# Autodesk Inventor part: Shaft
Saved by Autodesk Inventor 2014 (Build 180170000, 170)
## iProperties
Created: 2014-08-25
Part Number: Shaft
Material: Steel
Document SubType Name: Modeling
Designer: sam
Density: 1 g/cm^3
Appearance: Steel
CustomPartVersion: 1
Author: sam
Autodesk Inventor part; units mm, degrees
ref_plane "Start Plane" through (0, 0, 0) normal (1, 0, 0) x (0, 1, 0)
ref_plane "XZ Plane" through (0, 0, 0) normal (0, 1, 0) x (-1, 0, 0)
ref_plane "XY Plane" through (0, 0, 0) normal (0, 0, 1) x (1, 0, 0)
sketch "Main Sketch" plane through (0, 0, 0) normal (0, 0, 1) x (1, 0, 0)
  line L0 (0, 0) -> (10, 0)
  line L1 (0, 0) -> (0, 5.912)
  line L2 (0, 5.912) -> (5, 5.912)
  line L3 (10, 5.912) -> (10, 0)
  line L4 (5, 5.912) -> (10, 5.912)
  dimension "d3" = 11.824
  dimension "d4" = 11.824
  constraints: 10 end point, 4 horizontal, 2 vertical
  measures "d3" diameter of L2 L0
  measures "d4" diameter of L4 L0
revolve "Revolution1" add sketch "Main Sketch" angle 360 about axis through (0, 0, 0) along (1, 0, 0)
body "Solid1"
